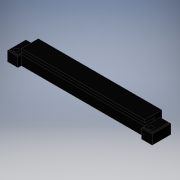
# Autodesk Inventor part: QSevenConnector
Saved by Autodesk Inventor 2016 (Build 200138000, 138)
## iProperties
Created: 2017-03-02
Part Number: QSevenConnector
Material: Generic
Document SubType Name: Modeling
Designer: jfixelle
Density: 1 g/cm^3
Appearance: Smooth - Black
Author: jfixelle
Autodesk Inventor part; units mm, degrees
ref_plane "YZ Plane" through (0, 0, 0) normal (1, 0, 0) x (0, 1, 0)
ref_plane "XZ Plane" through (0, 0, 0) normal (0, 1, 0) x (-1, 0, 0)
ref_plane "XY Plane" through (0, 0, 0) normal (0, 0, 1) x (1, 0, 0)
sketch "Sketch1" plane through (0, 0, 0) normal (0, 1, 0) x (-1, 0, 0)
  line L0 (32.355, 4.45) -> (-32.355, 4.45)
  line L1 (-32.355, 4.45) -> (-32.355, -4.45)
  line L2 (-32.355, -4.45) -> (32.355, -4.45)
  line L3 (32.355, -4.45) -> (32.355, 4.45)
  point P0 (0, 0)
  dimension "d0" = 64.71
  dimension "d1" = 32.355
  dimension "d2" = 8.9
  dimension "d3" = 4.45
  constraints: 8 end point, 2 parallel, 1 horizontal, 1 perpendicular
  measures "d0" distance of L1.end L2.end
  measures "d1" distance from line of point (0, 0) L3
  measures "d2" distance of L2.end L0.start
  measures "d3" distance from line of L2 point (0, 0)
extrude "Extrusion1" add sketch "Sketch1" along normal blind 7.8
sketch "Sketch2" plane through (0, 0, 0) normal (0, 1, 0) x (-1, 0, 0)
  line L0 (-32.355, 4.45) -> (-32.355, -4.45) projected
  line L1 (-32.355, -3.45) -> (-37.945, -3.45)
  line L2 (-37.945, -3.45) -> (-37.945, 6.25)
  line L3 (-37.945, 6.25) -> (-32.355, 6.25)
  line L4 (-32.355, 6.25) -> (-32.355, -3.45)
  line L5 (-32.355, -4.45) -> (32.355, -4.45) projected
  line L6 (32.355, -4.45) -> (32.355, 4.45) projected
  line L7 (32.355, -3.45) -> (37.855, -3.45)
  line L8 (37.855, -3.45) -> (37.855, 6.25)
  line L9 (37.855, 6.25) -> (32.355, 6.25)
  line L10 (32.355, 6.25) -> (32.355, -3.45)
  point P0 (0, 0)
  dimension "d6" = 10.7
  dimension "d7" = 5.59
  dimension "d8" = 10.7
  dimension "d9" = 5.5
  dimension "d10" = 1
  dimension "d11" = 1
  constraints: 16 end point, 4 parallel, 2 horizontal, 2 perpendicular, 2 point on line
  measures "d6" distance between parallel lines of L3 L5
  measures "d7" distance of L2.end L3.end
  measures "d8" distance between parallel lines of L5 L9
  measures "d9" distance of L8.end L9.end
  measures "d10" distance between parallel lines of L5 L1
  measures "d11" distance between parallel lines of L5 L7
extrude "Extrusion2" add sketch "Sketch2" along normal blind 5
sketch "Sketch3" plane through (-32.355, 7.8, 4.45) normal (0, 0, 1) x (1, 0, 0)
  line L0 (0, -2.8) -> (0, 0) projected
  line L1 (64.71, -7.8) -> (64.71, 0) projected
  line L2 (0, -2.8) -> (64.71, -2.8)
  line L3 (64.71, -2.8) -> (64.71, -1.35)
  line L4 (64.71, -1.35) -> (0, -1.35)
  line L5 (0, -1.35) -> (0, -2.8)
  point P0 (32.355, -7.8)
  dimension "d14" = 1.45
  constraints: 8 end point, 2 parallel, 1 horizontal, 1 perpendicular, 1 point on line
  measures "d14" distance between parallel lines of L2 L4
extrude "Extrusion3" cut sketch "Sketch3" against normal blind 5
sketch "Sketch4" plane through (0, 5, 0) normal (0, 1, 0) x (1, 0, 0)
  line L0 (32.355, -6.25) -> (37.945, -6.25) projected
  line L1 (37.945, 3.45) -> (32.355, 3.45) projected
  line L2 (37.945, -6.25) -> (32.355, -6.25)
  line L3 (32.355, -6.25) -> (32.355, 3.45)
  line L4 (32.355, 3.45) -> (37.945, 3.45)
  line L5 (37.945, 3.45) -> (37.945, -6.25)
  line L6 (-37.855, -6.25) -> (-32.355, -6.25) projected
  line L7 (-32.355, 3.45) -> (-37.855, 3.45) projected
  line L8 (-37.855, -6.25) -> (-32.355, -6.25)
  line L9 (-32.355, -6.25) -> (-32.355, 3.45)
  line L10 (-32.355, 3.45) -> (-37.855, 3.45)
  line L11 (-37.855, 3.45) -> (-37.855, -6.25)
  line L12 (-37.355, -5.75) -> (-32.855, -5.75)
  line L13 (-32.855, -5.75) -> (-32.855, 2.95)
  line L14 (-32.855, 2.95) -> (-37.355, 2.95)
  line L15 (-37.355, 2.95) -> (-37.355, -5.75)
  line L16 (32.855, -5.75) -> (37.445, -5.75)
  line L17 (37.445, -5.75) -> (37.445, 2.95)
  line L18 (37.445, 2.95) -> (32.855, 2.95)
  line L19 (32.855, 2.95) -> (32.855, -5.75)
  point P0 (0, 0)
  dimension "d17" = 0.5
  dimension "d18" = 0.5
  constraints: 32 end point, 8 parallel, 4 perpendicular, 2 horizontal, 6 other
  measures "d17" distance between parallel lines of L5 L17
  measures "d18" distance between parallel lines of L11 L15
extrude "Extrusion4" add sketch "Sketch4" along normal blind 0.5 contours L15 L14 L13 L12 | L19 L18 L17 L16
sketch "Sketch5" plane through (0, 5.5, 0) normal (0, 1, 0) x (1, 0, 0)
  circle A0 centre (35.205, -4.05) radius 1.15
  circle A1 centre (-35.205, -4.1) radius 1.15
  point P0 (0, 0)
  dimension "d21" = 4.1
  dimension "d22" = 4.05
  dimension "d23" = 70.41
  dimension "d24" = 35.205
  dimension "d35" = 2.3
  dimension "d36" = 2.3
  constraints: 2 centre point
  measures "d21" vertical distance of point (0, 0) A1.centre
  measures "d22" vertical distance of point (0, 0) A0.centre
  measures "d23" distance of A1.centre A0.centre
  measures "d24" horizontal distance of point (0, 0) A0.centre
  measures "d35" diameter of A1
  measures "d36" diameter of A0
extrude "Extrusion5" cut sketch "Sketch5" against normal through all
sketch "Sketch6" plane through (0, 0, 0) normal (0, -1, 0) x (1, 0, 0)
  circle A0 centre (30.75, 0) radius 0.75
  circle A1 centre (-30.75, 0) radius 0.75
  point P0 (0, 0)
  dimension "d27" = 61.5
  dimension "d28" = 30.75
  dimension "d29" = 1.5
  dimension "d30" = 1.5
  dimension "d33" = 0
  dimension "d34" = 0
  constraints: 2 centre point
  measures "d27" distance of A1.centre A0.centre
  measures "d28" distance of point (0, 0) A0.centre
  measures "d29" diameter of A0
  measures "d30" diameter of A1
  measures "d33" vertical distance of point (0, 0) A1.centre
  measures "d34" vertical distance of point (0, 0) A0.centre
extrude "Extrusion6" add sketch "Sketch6" along normal blind 1
body "Solid1"
